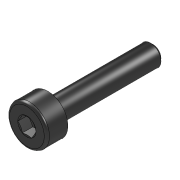
# Autodesk Inventor part: 10_053_CAP_BOLT_M2X10_R1
Saved by Autodesk Inventor 2021.2 (Build 252289000, 289)
## iProperties
Created: 2020-05-08
Part Number: 10_053_CAP_BOLT_M2X10_R1
Material: 鋼、炭素鋼
Document SubType Name: Modeling
Designer: y6tada
Density: 7.85 g/cm^3
Appearance: 光沢 - 黒
Author: y6tada
Autodesk Inventor part; units mm, degrees
ref_plane "YZ Plane" through (0, 0, 0) normal (1, 0, 0) x (0, 1, 0)
ref_plane "XZ Plane" through (0, 0, 0) normal (0, 1, 0) x (-1, 0, 0)
ref_plane "XY Plane" through (0, 0, 0) normal (0, 0, 1) x (1, 0, 0)
sketch "スケッチ1" plane through (0, 0, 0) normal (1, 0, 0) x (0, 1, 0)
  line L0 (0, 0) -> (1, 0) construction
  line L1 (1.9, 0) -> (1.9, 1.75)
  line L2 (1.65, 2) -> (0.866, 2)
  line L3 (0, 2) -> (0, 1.5) construction
  line L4 (1, 0) -> (1, -10)
  line L5 (1, -10) -> (0, -10)
  line L6 (0, -10) -> (0, 0)
  line L7 (1, 0) -> (1.9, 0)
  line L8 (0.866, 2) -> (0.433, 1.25) construction
  line L9 (0.433, 1.25) -> (-0.433, 1.25) construction
  line L10 (-0.433, 1.25) -> (-0.866, 2) construction
  line L11 (-0.866, 2) -> (-0.433, 2.75) construction
  line L12 (-0.433, 2.75) -> (0.433, 2.75) construction
  line L13 (0.433, 2.75) -> (0.866, 2) construction
  line L14 (0.866, 2) -> (0, 1.5)
  line L15 (0.866, 2) -> (0, 2) construction
  line L16 (0, 1.5) -> (0, 0)
  arc A0 (1.9, 1.75) -> (1.65, 2) centre (1.65, 1.75) ccw
  dimension "d0" = 1.5
  dimension "d1" = 3.8
  dimension "d2" = 2
  dimension "d3" = 10
  dimension "d4" = 2
  dimension "d6" = 0.25
  dimension "d11" = 30
  constraints: 34 end point, 7 parallel, 3 perpendicular, 2 horizontal, 2 point on circle, 2 tangent, 1 centre point, 1 coincident, 13 other
  measures "d0" distance between parallel lines of L9 L12
  measures "d1" diameter of L1 L3
  measures "d2" diameter of L4 L3
  measures "d3" distance of L0.end L4.end
  measures "d4" distance between parallel lines of L0 L2
  measures "d6" radius of A0
  measures "d11" angle of L15 L14
revolve "回転1" add sketch "スケッチ1" angle 360 about axis through (0, 0, 1.5) along (0, 0, -1)
sketch "スケッチ2" plane through (0, 0, 2) normal (0, 0, 1) x (1, 0, 0)
  line L0 (0.866, 0) -> (0.433, -0.75)
  line L1 (0.433, -0.75) -> (-0.433, -0.75)
  line L2 (-0.433, -0.75) -> (-0.866, 0)
  line L3 (-0.866, 0) -> (-0.433, 0.75)
  line L4 (-0.433, 0.75) -> (0.433, 0.75)
  line L5 (0.433, 0.75) -> (0.866, 0)
  point P0 (0, 0)
  point P1 (0, 0)
  dimension "d8" = 1.5
  constraints: 12 end point, 1 coincident, 1 horizontal, 13 other
  measures "d8" distance between parallel lines of L4 L1
extrude "押し出し1" cut sketch "スケッチ2" against normal blind 1
chamfer "面取り1" distance 0.25 angle 45 1 edges at (0, -1, -10)
